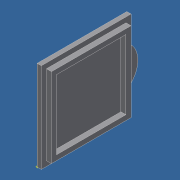
# Autodesk Inventor part: Modul Deckel
Saved by Autodesk Inventor 2018.2 (Build 222227000, 227)
## iProperties
Created: 2018-10-15
Part Number: Modul Deckel
Material: geeigneten Werkstoff auswählen !
Document SubType Name: Modeling
Designer: N.Grubert
Density: 0.001 g/cm^3
Appearance: Vorgabe
Author: N.Grubert
Fläche: 0 cm²
Gewicht: 0 g
Dateiname: P:\INVENTOR\Inventor 2018\Templates\ILT\Norm.ipt
Bez_eng: bolt
Bez_french: boulon
Autodesk Inventor part; units mm, degrees
ref_plane "YZ Plane" through (0, 0, 0) normal (1, 0, 0) x (0, 1, 0)
ref_plane "XZ Plane" through (0, 0, 0) normal (0, 1, 0) x (-1, 0, 0)
ref_plane "XY Plane" through (0, 0, 0) normal (0, 0, 1) x (1, 0, 0)
sketch "Skizze4" plane through (0, 0, 0) normal (1, 0, 0) x (0, 1, 0)
  line L0 (0, -10.6) -> (0, 63.6) construction
  line L1 (-10.6, 0) -> (63.6, 0) construction
  line L2 (53, 53) -> (0, 53)
  line L3 (0, 53) -> (0, 0)
  line L4 (0, 0) -> (53, 0)
  line L5 (53, 0) -> (53, 53)
  dimension "d4" = 53
  dimension "d5" = 53
  constraints: 8 end point, 2 parallel, 1 horizontal, 1 perpendicular
  measures "d4" distance between parallel lines of L0 L5
  measures "d5" distance between parallel lines of L2 L1
extrude "Extrusion2" add sketch "Skizze4" along normal blind 2.5
sketch "Skizze5" plane through (2.5, 0, 0) normal (1, 0, 0) x (0, 0, -1)
  line L0 (-53, 0) -> (0, 0) construction
  line L1 (0, 0) -> (0, 53) construction
  line L2 (0, 53) -> (-53, 53) construction
  line L3 (-53, 53) -> (-53, 0) construction
  line L4 (-50, 50) -> (-3, 50)
  line L5 (-3, 50) -> (-3, 3)
  line L6 (-3, 3) -> (-50, 3)
  line L7 (-50, 3) -> (-50, 50)
  line L8 (-6, 47) -> (-47, 47)
  line L9 (-47, 47) -> (-47, 6)
  line L10 (-47, 6) -> (-6, 6)
  line L11 (-6, 6) -> (-6, 47)
  dimension "d8" = 3
  dimension "d9" = 3
  constraints: 16 end point, 6 other
  measures "d8" distance between parallel lines of L2 L4
  measures "d9" distance between parallel lines of L4 L8
extrude "Extrusion3" add sketch "Skizze5" along normal blind 3
sketch "Skizze6" plane through (0, 0, 0) normal (-1, 0, 0) x (0, 0, 1)
  line L0 (53, 53) -> (0, 53) construction
  line L1 (53, 0) -> (53, 53) construction
  line L2 (0, 53) -> (0, 0) construction
  line L3 (26.5, 21.105) -> (26.5, 65.8226) construction
  line L4 (0, 53) -> (53, 53) projected
  arc A0 (37.2474, 53) -> (17.6514, 53) centre (27.4494, 43) ccw
  dimension "d12" = 26.5
  dimension "d13" = 53
  dimension "d14" = 14
  dimension "d15" = 10
  constraints: 2 end point, 2 point on circle, 2 point on line, 1 centre point, 1 vertical
  measures "d12" distance between parallel lines of L3 L1
  measures "d13" distance of L0.start L0.end
  measures "d14" radius of A0
  measures "d15" distance from line of A0.centre L0
extrude "Extrusion4" add sketch "Skizze6" against normal up to surface (2.5 mm away)
equation "\"d5\" = d4"
equation "\"d12\" = 0.5 * d13"
